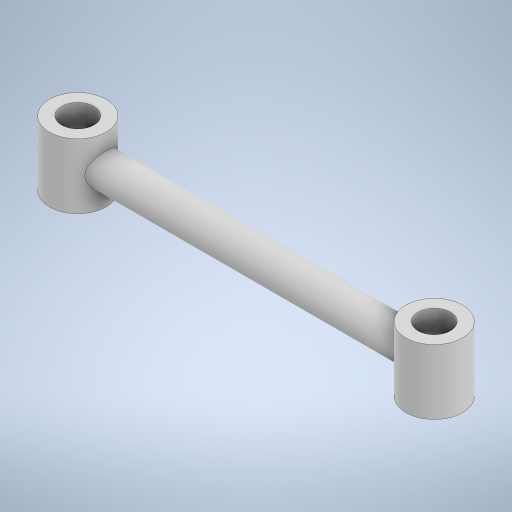
# Autodesk Inventor part: Part4
Saved by Autodesk Inventor 2024 (Build 280153000, 153)
## iProperties
Created: 2023-10-11
Part Number: Part4
Material: Generic
Document SubType Name: Modeling
Designer: owner
Density: 1 g/cm^3
Appearance: Default
Author: owner
Autodesk Inventor part; units mm, degrees
ref_plane "YZ Plane" through (0, 0, 0) normal (1, 0, 0) x (0, 1, 0)
ref_plane "XZ Plane" through (0, 0, 0) normal (0, 1, 0) x (-1, 0, 0)
ref_plane "XY Plane" through (0, 0, 0) normal (0, 0, 1) x (1, 0, 0)
sketch "Sketch1" plane through (0, 0, 0) normal (0, 0, 1) x (1, 0, 0)
  line L0 (0, 23.3412) -> (0, 0) construction
  line L1 (-110, 0) -> (0, 0)
  line L2 (110, 0) -> (0, 0)
  line L3 (-110, 0) -> (-110, 10)
  line L4 (-110, 10) -> (110, 10)
  line L5 (110, 10) -> (110, 0)
  dimension "d0" = 220
  dimension "d1" = 10
  constraints: 12 end point, 2 perpendicular, 2 vertical, 1 horizontal, 1 symmetric about line
  measures "d0" distance of L1.start L2.start
  measures "d1" distance of L4.end L2.start
revolve "Revolution1" add sketch "Sketch1" angle 360 about axis through (110, 0, 0) along (-1, 0, 0)
sketch "Sketch2" plane through (0, 0, 0) normal (0, 1, 0) x (-1, 0, 0)
  line L0 (110, -10) -> (110, 10) projected
  circle A0 centre (110, 0) radius 17.5
  circle A1 centre (110, 0) radius 10
  point P0 (0, 0)
  dimension "d3" = 20
  dimension "d4" = 35
  constraints: 2 centre point, 1 coincident, 1 midpoint
  measures "d3" diameter of A1
  measures "d4" diameter of A0
extrude "Extrusion1" add sketch "Sketch2" along normal mid plane 40 contours A1 L0 | L0 A1 | A0
extrude "Extrusion2" cut sketch "Sketch2" along normal mid plane 40 contours A1 L0 | L0 A1
mirror "Mirror1" about plane through (0, 0, 0) normal (1, 0, 0) of "Extrusion1"
sketch "Sketch3" plane through (110, 20, 0) normal (0, 1, 0) x (1, 0, 0)
  circle A0 centre (0, 0) radius 10
  circle A1 centre (0, 0) radius 17.5 projected
  point P0 (-110, 0)
  dimension "d9" = 20
  constraints: 1 centre point, 1 concentric
  measures "d9" diameter of A0
extrude "Extrusion3" cut sketch "Sketch3" against normal blind 40 contours A0
body "Solid1"
